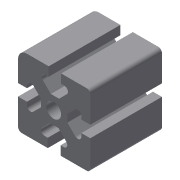
# Autodesk Inventor part: kylestslot
Saved by Autodesk Inventor 2015 (Build 190159000, 159)
## iProperties
Created: 2015-03-05
Part Number: kylestslot
Material: Generic
Document SubType Name: Modeling
Designer: Kyle
Density: 1 g/cm^3
Appearance: Default
Author: Kyle
Autodesk Inventor part; units mm, degrees
ref_plane "YZ Plane" through (0, 0, 0) normal (1, 0, 0) x (0, 1, 0)
ref_plane "XZ Plane" through (0, 0, 0) normal (0, 1, 0) x (-1, 0, 0)
ref_plane "XY Plane" through (0, 0, 0) normal (0, 0, 1) x (1, 0, 0)
sketch "Sketch1" plane through (0, 0, 0) normal (0, 0, 1) x (1, 0, 0)
  circle A0 centre (0, 0) radius 2.6035
  line L0 (0.3297, 4.515) -> (1.8944, 4.515)
  line L1 (4.8382, 1.3026) -> (4.8382, -0.0642)
  line L2 (4.8382, -0.0642) -> (4.8382, -1.3419)
  line L3 (4.8382, -0.0642) -> (6.1159, -0.0642) construction
  line L4 (1.6632, -4.5854) -> (0, -4.5854)
  line L5 (0, -4.5854) -> (-1.4104, -4.5854)
  line L6 (-4.5212, -1.3462) -> (-4.5212, 0)
  line L7 (-4.5212, 0) -> (-4.5212, 1.3026)
  line L8 (-1.0165, 4.515) -> (0.3297, 4.515)
  line L9 (1.8944, 4.515) -> (10.2327, 4.515) construction
  line L10 (1.8944, 4.515) -> (4.6655, 7.2861)
  line L11 (1.8944, 4.515) -> (5.8133, 4.515) construction
  line L12 (4.8382, 1.3026) -> (7.6093, 4.0737)
  line L13 (-1.0165, 4.515) -> (-3.7876, 7.2861)
  line L14 (-4.5212, 1.3026) -> (-7.2923, 4.0737)
  line L15 (-4.5212, -1.3462) -> (-7.2923, -4.1173)
  line L16 (-1.4104, -4.5854) -> (-4.1173, -7.2923)
  line L17 (1.6632, -4.5854) -> (4.4343, -7.3565)
  line L18 (4.8382, -1.3419) -> (7.6093, -4.113)
  line L19 (4.8382, -1.3419) -> (8.7572, -1.3419) construction
  line L20 (-2.8896, 9.4541) -> (-1.7646, 9.4541)
  line L21 (3.7675, 9.4541) -> (2.6425, 9.4541)
  line L22 (-9.4603, 3.1757) -> (-9.4603, 2.0507)
  line L23 (-9.4603, -3.2193) -> (-9.4603, -2.0943)
  line L24 (-3.2193, -9.4603) -> (-2.0943, -9.4603)
  line L25 (3.5363, -9.5246) -> (2.4114, -9.5246)
  line L26 (9.7774, -3.215) -> (9.7774, -2.0901)
  line L27 (9.7774, 3.1757) -> (9.7774, 2.0507)
  line L28 (-1.7646, 9.4541) -> (-1.7646, 12.6291)
  line L29 (-9.4603, 2.0507) -> (-12.6353, 2.0507)
  line L30 (-9.4603, -2.0943) -> (-12.6353, -2.0943)
  line L31 (-2.0943, -9.4603) -> (-2.0943, -12.6353)
  line L32 (2.4114, -9.5246) -> (2.4114, -12.6996)
  line L33 (9.7774, -2.0901) -> (12.9524, -2.0901)
  line L34 (9.7774, 2.0507) -> (12.9524, 2.0507)
  line L35 (2.6425, 9.4541) -> (2.6425, 12.6291)
  line L36 (-1.7646, 12.6291) -> (-9.4603, 12.6291)
  line L37 (-12.6353, 9.4541) -> (-12.6353, 2.0507)
  line L38 (-12.6353, -2.0943) -> (-12.6353, -11.3653)
  line L39 (-11.3653, -12.6353) -> (-2.0943, -12.6353)
  line L40 (12.9524, -2.0901) -> (12.9524, -11.4296)
  line L41 (11.6824, -12.6996) -> (2.4114, -12.6996)
  line L42 (12.9524, 2.0507) -> (12.9524, 11.3591)
  line L43 (11.6824, 12.6291) -> (2.6425, 12.6291)
  arc A1 (-9.4603, 12.6291) -> (-12.6353, 9.4541) centre (-9.4603, 9.4541) ccw
  arc A2 (-2.8896, 9.4541) -> (-3.7876, 7.2861) centre (-2.8896, 8.1841) ccw
  arc A3 (-7.2923, 4.0737) -> (-9.4603, 3.1757) centre (-8.1903, 3.1757) ccw
  arc A4 (-9.4603, -3.2193) -> (-7.2923, -4.1173) centre (-8.1903, -3.2193) ccw
  arc A5 (-4.1173, -7.2923) -> (-3.2193, -9.4603) centre (-3.2193, -8.1903) ccw
  arc A6 (3.5363, -9.5246) -> (4.4343, -7.3565) centre (3.5363, -8.2546) ccw
  arc A7 (7.6093, -4.113) -> (9.7774, -3.215) centre (8.5074, -3.215) ccw
  arc A8 (9.7774, 3.1757) -> (7.6093, 4.0737) centre (8.5074, 3.1757) ccw
  arc A9 (4.6655, 7.2861) -> (3.7675, 9.4541) centre (3.7675, 8.1841) ccw
  arc A10 (12.9524, 11.3591) -> (11.6824, 12.6291) centre (11.6824, 11.3591) ccw
  arc A11 (11.6824, -12.6996) -> (12.9524, -11.4296) centre (11.6824, -11.4296) ccw
  arc A12 (-12.6353, -11.3653) -> (-11.3653, -12.6353) centre (-11.3653, -11.3653) ccw
  point P0 (4.8382, 4.515)
  point P1 (4.8382, -4.5854)
  point P2 (-4.5212, -4.5854)
  point P3 (-4.5212, 4.515)
  point P4 (6.8335, 9.4541)
  point P5 (9.7774, 6.2417)
  point P6 (-5.9556, 9.4541)
  point P7 (-9.4603, 6.2417)
  point P8 (-9.4603, -6.2853)
  point P9 (-6.2853, -9.4603)
  point P10 (6.6024, -9.5246)
  point P11 (9.7774, -6.2811)
  dimension "d0" = 5.207
  dimension "d1" = 4.5085
  dimension "d2" = 90
  dimension "d3" = 4.5212
  dimension "d4" = 90
  dimension "d5" = 4.5212
  dimension "d9" = 6.985
  dimension "d10" = 45
  dimension "d11" = 6.985
  dimension "d12" = 6.985
  dimension "d13" = 6.985
  dimension "d14" = 6.985
  dimension "d15" = 6.985
  dimension "d16" = 6.985
  dimension "d17" = 45
  dimension "d18" = 4.191
  dimension "d19" = 4.191
  dimension "d20" = 4.191
  dimension "d21" = 4.191
  dimension "d22" = 4.191
  dimension "d23" = 4.191
  dimension "d24" = 4.191
  dimension "d25" = 4.191
  dimension "d26" = 3.175
  dimension "d27" = 3.175
  dimension "d28" = 3.175
  dimension "d29" = 3.175
  dimension "d30" = 3.175
  dimension "d31" = 1.27
  dimension "d32" = 1.27
  constraints: 88 end point, 26 point on line, 24 point on circle, 24 tangent, 16 horizontal, 13 centre point, 10 vertical, 9 equal radius, 6 perpendicular, 3 equal length, 1 coincident, 1 collinear
  measures "d0" diameter of A0
  measures "d1" distance of L0.start point (4.838, 4.515)
  measures "d2" angle of L0 L1
  measures "d3" distance of L1.end point (4.838, -4.585)
  measures "d4" angle of L2 L3
  measures "d5" distance of L4.end point (-4.521, -4.585)
  measures "d9" distance of L0.end point (6.834, 9.454)
  measures "d10" angle of L11 L10
  measures "d11" distance of L1.start point (9.777, 6.242)
  measures "d12" distance of L8.start point (-5.956, 9.454)
  measures "d13" distance of L7.end point (-9.46, 6.242)
  measures "d14" distance of L6.start point (-9.46, -6.285)
  measures "d15" distance of L4.start point (6.602, -9.525)
  measures "d16" distance of L2.end point (9.777, -6.281)
  measures "d17" angle of L18 L19
  measures "d18" distance of point (-5.956, 9.454) L20.end
  measures "d19" distance of point (6.834, 9.454) L21.end
  measures "d20" distance of point (-9.46, 6.242) L22.end
  measures "d21" distance of point (-9.46, -6.285) L23.end
  measures "d22" distance of point (-6.285, -9.46) L24.end
  measures "d23" distance of point (6.602, -9.525) L25.end
  measures "d24" distance of point (9.777, -6.281) L26.end
  measures "d25" distance of point (9.777, 6.242) L27.end
  measures "d26" distance of L20.end L28.end
  measures "d27" distance of L22.end L29.end
  measures "d28" distance of L24.end L31.end
  measures "d29" distance of L26.end L33.end
  measures "d30" radius of A1
  measures "d31" radius of A2
  measures "d32" radius of A8
extrude "Extrusion1" add sketch "Sketch1" along normal blind 25.4
body "Solid1"
